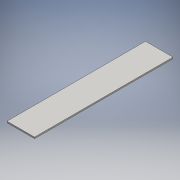
# Autodesk Inventor part: filter base
Saved by Autodesk Inventor 2016 SP1 (Build 200210100, 210)
## iProperties
Created: 2016-05-25
Part Number: filter base
Material: Rubber
Document SubType Name: Modeling
Designer: ubik
Density: 0.93 g/cm^3
Appearance: Rubber - Black
Author: ubik
Autodesk Inventor part; units mm, degrees
ref_plane "YZ Plane" through (0, 0, 0) normal (1, 0, 0) x (0, 1, 0)
ref_plane "XZ Plane" through (0, 0, 0) normal (0, 1, 0) x (-1, 0, 0)
ref_plane "XY Plane" through (0, 0, 0) normal (0, 0, 1) x (1, 0, 0)
sketch "Sketch1" plane through (0, 0, 0) normal (0, 0, 1) x (1, 0, 0)
  line L0 (-28.5, 143.5) -> (28.5, 143.5)
  line L1 (28.5, 143.5) -> (28.5, -143.5)
  line L2 (28.5, -143.5) -> (-28.5, -143.5)
  line L3 (-28.5, -143.5) -> (-28.5, 143.5)
  point P0 (0, 0)
  dimension "d0" = 57
  dimension "d1" = 287
  dimension "d2" = 143.5
  dimension "d3" = 28.5
  constraints: 8 end point, 2 parallel, 1 horizontal, 1 perpendicular
  measures "d0" distance of L0.start L0.end
  measures "d1" distance of L2.end L0.start
  measures "d2" distance from line of point (0, 0) L0
  measures "d3" distance from line of point (0, 0) L3
extrude "Extrusion1" add sketch "Sketch1" along normal blind 3
equation "\"d2\" = 0.5 * d1"
equation "\"d3\" = 0.5 * d0"
body "Solid1"
